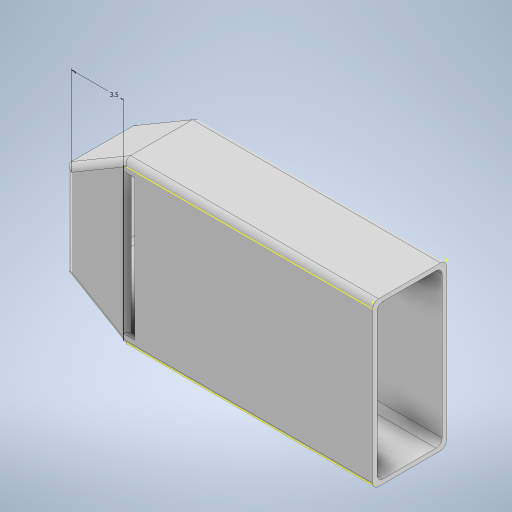
# Autodesk Inventor part: np2_headstage_box
Saved by Autodesk Inventor 2023.3 (Build 273359000, 359)
## iProperties
Created: 2023-11-21
Part Number: np2_headstage_box
Material: Generic
Document SubType Name: Modeling
Designer: mmelin
Density: 1 g/cm^3
Appearance: Default
Author: mmelin
Autodesk Inventor part; units mm, degrees
ref_plane "YZ Plane" through (0, 0, 0) normal (1, 0, 0) x (0, 1, 0)
ref_plane "XZ Plane" through (0, 0, 0) normal (0, 1, 0) x (-1, 0, 0)
ref_plane "XY Plane" through (0, 0, 0) normal (0, 0, 1) x (1, 0, 0)
sketch "Sketch1" plane through (0, 0, 0) normal (0, 0, 1) x (1, 0, 0)
  line L0 (0, -11) -> (-16.777, -11)
  line L1 (-16.777, -11) -> (-16.777, -10.7)
  line L2 (-16.777, -10.7) -> (0, -10.7)
  line L3 (0, -10.7) -> (0, -11)
  line L4 (0, -0.3) -> (-16.777, -0.3)
  line L5 (-16.777, -0.3) -> (-16.777, 0)
  line L6 (-16.777, 0) -> (0, 0)
  line L7 (0, 0) -> (0, -0.3)
  line L8 (-20.377, -8.65) -> (-20.777, -8.65)
  line L9 (-20.777, -8.65) -> (-20.777, -2.35)
  line L10 (-20.777, -2.35) -> (-20.377, -2.35)
  line L11 (-20.377, -2.35) -> (-20.377, -8.65)
  line L12 (-20.377, -8.65) -> (-16.777, -10.7)
  line L13 (-16.777, -11) -> (-20.777, -8.65)
  line L14 (-20.777, -2.35) -> (-16.777, 0)
  line L15 (-20.377, -2.35) -> (-16.777, -0.3)
  dimension "d0" = 0.3
  dimension "d2" = 10.4
  dimension "d3" = 0.4
  dimension "d4" = 4
  dimension "d21" = 20.777
  dimension "d22" = 6.3
  constraints: 32 end point, 6 parallel, 3 horizontal, 3 perpendicular, 2 equal length, 1 coincident, 1 collinear, 1 point on line
  measures "d0" distance of L2.end L0.start
  measures "d2" distance between parallel lines of L4 L2
  measures "d3" distance of L8.start L8.end
  measures "d4" distance between parallel lines of L9 L1
  measures "d21" distance between parallel lines of L9 L7
  measures "d22" distance between parallel lines of L8 L10
extrude "Extrusion1" add sketch "Sketch1" along normal blind 5
sketch "Sketch2" plane through (-16.777, -10.7, 0) normal (0, 1, 0) x (1, 0, 0)
  line L0 (4.777, -3.6) -> (4.377, -3.6)
  line L1 (4.377, -3.6) -> (4.377, -1.4)
  line L2 (4.377, -1.4) -> (4.777, -1.4)
  line L3 (4.777, -1.4) -> (4.777, -3.6)
  line L4 (4.777, -3.6) -> (4.777, -5) construction
  line L5 (16.777, -5) -> (0, -5) construction
  line L6 (4.777, -1.4) -> (4.777, 0) construction
  line L7 (16.777, 0) -> (0, 0) construction
  line L8 (16.777, 0) -> (16.777, -5) construction
  dimension "d9" = 0.4
  dimension "d10" = 1.4
  dimension "d11" = 12
  constraints: 12 end point, 3 point on line, 2 parallel, 1 collinear, 1 horizontal, 1 perpendicular, 1 vertical
  measures "d9" distance of L0.start L0.end
  measures "d10" distance of L2.end L6.end
  measures "d11" distance between parallel lines of L8 L3
extrude "Extrusion2" add sketch "Sketch2" along normal blind 0.5
sketch "Sketch3" plane through (-16.777, -0.3, 0) normal (0, -1, 0) x (1, 0, 0)
  line L0 (4.777, 1.4) -> (4.377, 1.4) projected
  line L1 (4.377, 1.4) -> (4.377, 3.6) projected
  line L2 (4.377, 3.6) -> (4.777, 3.6) projected
  line L3 (4.777, 3.6) -> (4.777, 1.4) projected
  point P0 (16.777, 0)
extrude "Extrusion3" add sketch "Sketch3" along normal blind 0.5
sketch "Sketch4" plane through (0, -0.3, 0) normal (1, 0, 0) x (0, 0, -1)
  line L0 (0, -10.4) -> (-5, -10.4) projected
  line L1 (0, 0) -> (-5, 0) projected
  line L2 (-5, -10.4) -> (-4.7, -10.4)
  line L3 (-4.7, -10.4) -> (-4.7, 0)
  line L4 (-4.7, 0) -> (-5, 0)
  line L5 (-5, 0) -> (-5, -10.4)
  line L6 (0, 0) -> (-0.3, 0)
  line L7 (-0.3, 0) -> (-0.3, -10.4)
  line L8 (-0.3, -10.4) -> (0, -10.4)
  line L9 (0, -10.4) -> (0, 0)
  point P0 (0, 0.3)
  point P1 (-0.3, 0)
  dimension "d16" = 0.3
  dimension "d17" = 0.3
  constraints: 16 end point, 4 parallel, 2 horizontal, 2 perpendicular, 2 point on line
  measures "d16" distance between parallel lines of L7 L9
  measures "d17" distance between parallel lines of L5 L3
extrude "Extrusion4" add sketch "Sketch4" against normal up to next contours L0 L7 L1 L9 | L0 L5 L1 L3
fillet "Fillet1" radius 0.4 18 edges at (-20.777, -5.5, 0) (-18.777, -9.825, 0) (-18.777, -9.825, 5) (-20.777, -5.5, 5) (-18.777, -1.175, 0) (-18.777, -1.175, 5) (-8.3885, 0, 5) (-8.3885, 0, 0) (-8.3885, -11, 5) (-8.3885, -11, 0) (-8.3885, -10.7, 0.3) (-16.777, -10.7, 2.5) (-20.377, -8.65, 2.5) (-20.377, -2.35, 2.5) (-16.777, -0.3, 2.5) (-8.3885, -0.3, 0.3) (-8.3885, -0.3, 4.7) (-8.3885, -10.7, 4.7)
sketch "Sketch5" plane through (0, 0, 5) normal (0, 0, 1) x (1, 0, 0)
  line L0 (0, -0.4) -> (-16.6682, -0.4) projected
  line L1 (-16.877, -0.4) -> (-16.877, -10.7)
  line L2 (-16.6711, -10.7) -> (0, -10.7) projected
  line L3 (-20.377, -8.4211) -> (-20.377, -2.5789) projected
  point P0 (0, 0)
  dimension "d23" = 3.5
  constraints: 2 end point, 2 point on line, 1 vertical
  measures "d23" distance between parallel lines of L3 L1
ref_plane "Work Plane1" through (-16.877, -0.4, 5) normal (-0.6427876, 0, 0.7660444) x (0, -1, 0)
sketch "Sketch6" plane through (0, 0, 0) normal (0, 0, -1) x (-1, 0, 0)
  line L0 (16.877, -0.4) -> (16.877, -10.7) projected
  point P0 (0, 0)
ref_plane "Work Plane2" through (-16.877, -0.4, 0) normal (-0.6427876, 0, -0.7660444) x (0, -1, 0)
sketch "Sketch7" plane through (-16.877, -0.4, 5) normal (-0.6427876, 0, 0.7660444) x (0, -1, 0)
  line L0 (0.35, 0.6) -> (9.85, 0.6)
  line L1 (9.85, 0.6) -> (9.85, 0)
  line L2 (9.85, 0) -> (0.35, 0)
  line L3 (0.35, 0) -> (0.35, 0.6)
  line L4 (0, 0) -> (10.3, 0) projected
  line L5 (-0.4, 12.6714) -> (-0.4, -0.1805) construction
  line L6 (10.6, -0.1805) -> (10.6, 12.6714) construction
  line L7 (0.35, 0.6) -> (-0.4, 0.6) construction
  line L8 (9.85, 0.6) -> (10.6, 0.6) construction
  point P0 (-0.4, 9.7146)
  dimension "d26" = 9.5
  dimension "d27" = 0.6
  constraints: 12 end point, 3 point on line, 2 collinear, 2 parallel, 2 perpendicular, 1 horizontal
  measures "d26" distance of L0.start L0.end
  measures "d27" distance of L2.end L0.start
extrude "Extrusion5" cut sketch "Sketch7" against normal blind 3
sketch "Sketch8" plane through (-16.877, -0.4, 0) normal (-0.6427876, 0, -0.7660444) x (0, -1, 0)
  line L0 (9.85, -0.6) -> (0.35, -0.6)
  line L1 (0.35, -0.6) -> (0.35, 0)
  line L2 (0.35, 0) -> (9.85, 0)
  line L3 (9.85, 0) -> (9.85, -0.6)
  line L4 (0, 0) -> (10.3, 0) projected
  line L5 (0.35, 3.2139) -> (0.35, 2.6139) projected
  line L6 (9.85, 2.6139) -> (9.85, 3.2139) projected
  line L7 (10.6, -12.6714) -> (10.6, 0.1805) projected
  line L8 (-0.4, 0.1805) -> (-0.4, -12.6714) projected
  line L9 (0.35, -0.6) -> (-0.4, -0.6) construction
  line L10 (9.85, -0.6) -> (10.6, -0.6) construction
  point P0 (-0.4, -12.9285)
  dimension "d30" = 9.5
  dimension "d31" = 0.6
  constraints: 12 end point, 3 point on line, 2 collinear, 2 parallel, 2 perpendicular, 1 horizontal
  measures "d30" distance of L0.start L0.end
  measures "d31" distance of L2.end L0.start
extrude "Extrusion6" cut sketch "Sketch8" against normal blind 3
equation "\"d17\" = d16"
body "Solid1"
